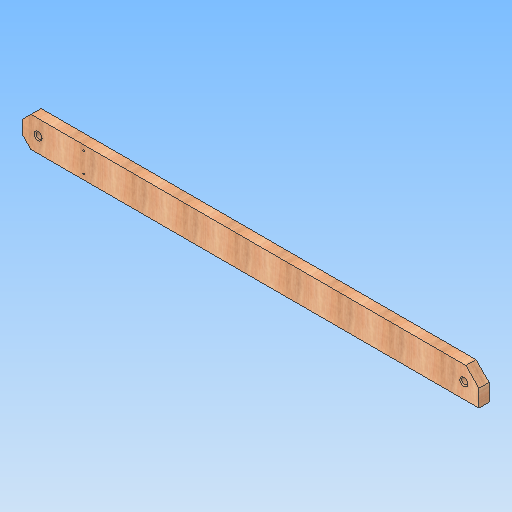
# Autodesk Inventor part: Top_Rear Plank_LHS
Saved by Autodesk Inventor 2018.1 (Build 221171000, 171)
## iProperties
Created: 2019-03-15
Part Number: Top_Rear Plank_LHS
Material: Wood (Birch)
Document SubType Name: Modeling
Designer: James
Density: 0.55 g/cm^3
Appearance: Birch - Natural Polished
Mass: 9134 g
Surface Area: 9112.98 cm^2
Volume: 16607.3 cm^3
Author: James
Autodesk Inventor part; units mm, degrees
ref_plane "YZ Plane" through (0, 0, 0) normal (1, 0, 0) x (0, 1, 0)
ref_plane "XZ Plane" through (0, 0, 0) normal (0, 1, 0) x (-1, 0, 0)
ref_plane "XY Plane" through (0, 0, 0) normal (0, 0, 1) x (1, 0, 0)
sketch "Sketch1" plane through (0, 0, 0) normal (0, 0, 1) x (1, 0, 0)
  line L0 (0, 0) -> (2250, 0)
  line L1 (2250, 0) -> (2250, 150)
  line L2 (2250, 150) -> (0, 150)
  line L3 (0, 150) -> (0, 0)
  dimension "d0" = 150
  dimension "d1" = 2250
  constraints: 8 end point, 2 parallel, 1 horizontal, 1 perpendicular
  measures "d0" distance of L0.end L1.end
  measures "d1" distance of L1.end L2.end
extrude "Extrusion1" add sketch "Sketch1" along normal blind 50
sketch "Sketch2" plane through (0, 0, 50) normal (0, 0, 1) x (1, 0, 0)
  line L0 (0, 150) -> (0, 0) projected
  line L1 (2250, 0) -> (2250, 150) projected
  point P0 (75, 75)
  point P1 (2175, 75)
  point P2 (0, 75)
  dimension "d4" = 75
  dimension "d5" = 75
  constraints: 2 horizontal alignment, 1 midpoint
  measures "d4" distance from line of point (75, 75) L0
  measures "d5" distance from line of L1 point (2175, 75)
hole "Hole1" at (75, 75, 50) at (2175, 75, 50) direction (0, 0, -1) diameter 30 end through all
chamfer "Chamfer1" distance 5 angle 45 4 edges at (75, 90, 50) (2175, 90, 50) (75, 90, 0) (2175, 90, 0)
chamfer "Chamfer2" distance 65 angle 45 1 edges at (2250, 150, 25) measured on face at (2250, 50, 16.6667)
chamfer "Chamfer3" distance 40 angle 45 2 edges at (0, 150, 25) (0, 0, 25)
sketch "Sketch3" plane through (0, 0, 0) normal (0, 0, -1) x (-1, 0, 0)
  line L0 (-40, 0) -> (-2250, 0) projected
  line L1 (-2185, 150) -> (-40, 150) projected
  line L2 (0, 110) -> (0, 40) projected
  point P0 (0, 0)
  point P1 (-300, 25)
  point P2 (-300, 125)
  dimension "d22" = 25
  dimension "d23" = 25
  dimension "d24" = 300
  constraints: 1 vertical alignment
  measures "d22" distance from line of L0 point (-300, 25)
  measures "d23" distance from line of L1 point (-300, 125)
  measures "d24" distance from line of point (-300, 25) L2
hole "Hole2" at (300, 25, 0) at (300, 125, 0) direction (0, 0, 1) diameter 8.433 end through all countersink diameter 16.129 countersink angle 82 clearance for "Flat Head Machine Screw (82)" size "5/16" standard "Ansi Unified Screw Threads"
equation "\"d23\" = d22"
body "Solid1"
